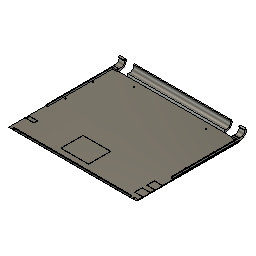
D_case (Autodesk Fusion 360 design; units mm, degrees)
Autodesk Fusion 360 part; units mm, degrees
sketch "Sketch2" plane through (0, 0, 0) normal (1, 0, 0) x (0, 0, -1)
  line L0 (0, 0) -> (0, 1.5)
  line L1 (0, 1.5) -> (190.1699, 1.5)
  line L2 (0, 0) -> (190.1699, 0)
  circle A0 centre (194.5, 12) radius 10.5
  circle A1 centre (194.5, 12) radius 9
  circle A2 centre (190.1699, 17.5) radius 17.5
  circle A3 centre (190.1699, 17.5) radius 16
  line L3 (203.5, 12) -> (205, 12)
  circle A4 centre (194.5, 12) radius 7.5
  line L4 (194.5, 12) -> (202.9853, 15)
  line L5 (194.5, 12) -> (190.1699, 1.5)
  dimension "d1" = 1.5
  dimension "d2" = 21
  dimension "d3" = 18
  dimension "d4" = 35
  dimension "d5" = 32
  dimension "d6" = 10.5
  dimension "d7" = 205
  dimension "d48" = 15
  dimension "d50" = 3
  constraint coincident L0.start L2.start
  constraint vertical L0
  constraint perpendicular L0 L1
  constraint perpendicular L0 L2
  constraint concentric A0 A1
  constraint tangent A0 A2
  constraint tangent L2 A2
  constraint coincident L2.end A2
  constraint concentric A2 A3
  constraint coincident L1.end A3
  constraint coincident A1 L3.start
  constraint coincident A0 L3.end
  constraint horizontal L3
  constraint tangent L1 A0
  constraint concentric A0 A4
  constraint coincident A0.centre A1.centre
  constraint coincident A1 L4.end
  measures "d1" distance of L0.start L0.end
  measures "d2" diameter of A0
  measures "d3" diameter of A1
  measures "d4" diameter of A2
  measures "d5" diameter of A3
  measures "d6" distance of L1 L3
  measures "d7" distance of L0 L3.end
  measures "d48" diameter of A4
  measures "d50" vertical distance of L3.start L4.end
extrude "Extrude1" add sketch "Sketch2" along normal blind 230.6 contours L0 L1 L2 A2 | L1 A0 A2 A3 | A0 A3 | A0 A3 L5 | A0 A1 A3 L5 | A0 A1 A3 L3 | A1 A4 L4 L5 picked at (191.2125, 0.5585) picked at (190.5457, 1.771) picked at (199.275, 4.984)
sketch "Sketch3" plane through (0, 0, 0) normal (0, -1, 0) x (1, 0, 0)
  line L0 (0, 0) -> (0, -190.1699)
  line L1 (0, -190.1699) -> (230.6, -190.1699)
  line L2 (230.6, -190.1699) -> (230.6, 0)
  line L3 (230.6, 0) -> (0, 0)
  circle A0 centre (6, -6) radius 6
  circle A1 centre (224.6, -6) radius 6
  line L4 (230.6, -6) -> (230.6, 0)
  line L5 (224.6, 0) -> (230.6, 0)
  line L6 (6, 0) -> (0, 0)
  line L7 (0, -6) -> (0, 0)
  dimension "d10" = 12
  dimension "d11" = 12
  constraint tangent L3 A0
  constraint tangent L0 A0
  constraint tangent L3 A1
  constraint tangent L2 A1
  constraint coincident A1 L4.start
  constraint coincident L2.end L3.start
  constraint tangent A1 L4
  constraint coincident A1 L5.start
  constraint tangent A1 L5
  constraint coincident A0 L6.start
  constraint coincident L0.start L3.end
  constraint perpendicular L0 L6
  constraint coincident A0 L7.start
  constraint perpendicular L6 L7
  measures "d10" diameter of A0
  measures "d11" diameter of A1
extrude "Extrude2" cut sketch "Sketch3" against normal through all contours L0 L3 A0 L6 L7 | L2 L3 A1 L4 L5
sketch "Sketch4" plane through (0, 0, 0) normal (0, -1, 0) x (1, 0, 0)
  arc A0 (6, 0) -> (0, -6) centre (6, -6) ccw
  line L0 (0, -6) -> (0, -190.1699)
  line L1 (0, -190.1699) -> (230.6, -190.1699)
  line L2 (230.6, -190.1699) -> (230.6, -6)
  arc A1 (230.6, -6) -> (224.6, 0) centre (224.6, -6) ccw
  line L3 (224.6, 0) -> (6, 0)
  line L4 (0, -190) -> (1.5, -190)
  line L5 (1.5, -190) -> (1.5, -215)
  line L6 (1.5, -215) -> (0, -215)
  line L7 (0, -215) -> (0, -190)
  line L8 (230.6, -190) -> (229.1, -190)
  line L9 (229.1, -190) -> (229.1, -215)
  line L10 (229.1, -215) -> (230.6, -215)
  line L11 (230.6, -215) -> (230.6, -190)
  line L12 (11.5, -190) -> (27.5, -190)
  line L13 (27.5, -190) -> (27.5, -215)
  line L14 (27.5, -215) -> (11.5, -215)
  line L15 (11.5, -215) -> (11.5, -190)
  line L16 (203.1, -190) -> (219.1, -190)
  line L17 (219.1, -190) -> (219.1, -215)
  line L18 (219.1, -215) -> (203.1, -215)
  line L19 (203.1, -215) -> (203.1, -190)
  dimension "d13" = 1.5
  dimension "d14" = 25
  dimension "d15" = 1.5
  dimension "d83" = 16
  dimension "d84" = 10
  dimension "d85" = 10
  dimension "d86" = 16
  dimension "d87" = 190
  constraint horizontal L4
  constraint vertical L5
  constraint horizontal L6
  constraint vertical L7
  constraint horizontal L8
  constraint vertical L9
  constraint horizontal L10
  constraint vertical L11
  constraint horizontal L12
  constraint vertical L13
  constraint horizontal L14
  constraint vertical L15
  constraint horizontal L16
  constraint vertical L17
  constraint horizontal L18
  constraint vertical L19
  constraint equal L5 L15
  constraint equal L13 L19
  constraint collinear L2 L11
  constraint collinear L0 L7
  constraint collinear L4 L12
  constraint collinear L12 L16
  constraint collinear L8 L16
  constraint equal L9 L17
  measures "d13" distance of L4.start L4.end
  measures "d14" distance of L4.start L6.end
  measures "d15" distance of L8.start L8.end
  measures "d83" distance of L13.end L14.end
  measures "d84" distance of L5 L15
  measures "d85" distance of L9 L17
  measures "d86" distance of L17.end L18.end
  measures "d87" distance of L3 L4
extrude "Extrude3" cut sketch "Sketch4" against normal through all contours L0 L1 L4 L5 L7 | L1 L5 L6 L7 | L1 L2 L8 L9 L11 | L1 L9 L10 L11 | L1 L12 L13 L15 | L1 L13 L14 L15 | L1 L17 L18 L19 | L1 L16 L17 L19
sketch "Sketch13" plane through (0, 1.5, 0) normal (0, 1, 0) x (-1, 0, 0)
  line L0 (0, -190) -> (0, -6)
  arc A0 (0, -6) -> (-6, 0) centre (-6, -6) ccw
  line L1 (-6, 0) -> (-224.6, 0)
  arc A1 (-224.6, 0) -> (-230.6, -6) centre (-224.6, -6) ccw
  line L2 (-230.6, -6) -> (-230.6, -190)
  line L3 (-230.6, -190) -> (-229.1, -190)
  line L4 (-229.1, -190) -> (-229.1, -190.1699)
  line L5 (-229.1, -190.1699) -> (-219.1, -190.1699)
  line L6 (-219.1, -190.1699) -> (-219.1, -190)
  line L7 (-219.1, -190) -> (-203.1, -190)
  line L8 (-203.1, -190) -> (-203.1, -190.1699)
  line L9 (-203.1, -190.1699) -> (-27.5, -190.1699)
  line L10 (-27.5, -190.1699) -> (-27.5, -190)
  line L11 (-27.5, -190) -> (-11.5, -190)
  line L12 (-11.5, -190) -> (-11.5, -190.1699)
  line L13 (-11.5, -190.1699) -> (-1.5, -190.1699)
  line L14 (-1.5, -190.1699) -> (-1.5, -190)
  line L15 (-1.5, -190) -> (0, -190)
  line L16 (-1.5, -188.1699) -> (-11.5, -188.1699)
  line L17 (-11.5, -188.1699) -> (-11.5, -192.1699)
  line L18 (-11.5, -192.1699) -> (-1.5, -192.1699)
  line L19 (-1.5, -192.1699) -> (-1.5, -188.1699)
  line L20 (-115.3, -219.4549) -> (-115.3, 20.5451) construction
  line L21 (-229.1, -188.1699) -> (-219.1, -188.1699)
  line L22 (-219.1, -188.1699) -> (-219.1, -192.1699)
  line L23 (-229.1, -192.1699) -> (-229.1, -188.1699)
  line L24 (-219.1, -192.1699) -> (-229.1, -192.1699)
  dimension "d90" = 2
  dimension "d91" = 4
  constraint horizontal L16
  constraint vertical L17
  constraint horizontal L18
  constraint vertical L19
  constraint collinear L12 L17
  constraint collinear L14 L19
  constraint perpendicular L1 L20
  constraint symmetric L16.start L20 L21.start
  constraint symmetric L16.end L20 L21.end
  constraint symmetric L17.end L20 L22.end
  constraint symmetric L18.end L20 L23.start
  measures "d90" distance of L13 L16
  measures "d91" distance of L16 L18
extrude "Extrude10" add sketch "Sketch13" along normal blind 3 contours L12 L13 L14 L16 L17 L19 | L13 L17 L18 L19 | L4 L5 L6 L21 L22 L23 | L5 L22 L23 L24
sketch "Sketch14" plane through (0, -50.4588, -17.8399) normal (0, 0.942809, 0.333333) x (1, 0, 0)
  line L0 (11.5, 194.8764) -> (11.5, 196.3764)
  line L1 (11.5, 196.3764) -> (1.5, 196.3764)
  line L2 (1.5, 196.3764) -> (1.5, 194.8764)
  line L3 (1.5, 194.8764) -> (11.5, 194.8764)
  line L4 (1.5, 196.3764) -> (11.5, 196.3764)
  line L5 (11.5, 196.3764) -> (11.5, 193.3764)
  line L6 (11.5, 193.3764) -> (1.5, 193.3764)
  line L7 (1.5, 193.3764) -> (1.5, 196.3764)
  line L8 (115.3, 222.5884) -> (115.3, -60) construction
  line L9 (0, 6.1569) -> (0, 179.6337)
  line L10 (230.6, 179.6337) -> (230.6, 6.1569)
  line L11 (229.1, 196.3764) -> (219.1, 196.3764)
  line L12 (219.1, 196.3764) -> (219.1, 193.3764)
  line L13 (219.1, 193.3764) -> (229.1, 193.3764)
  line L14 (229.1, 193.3764) -> (229.1, 196.3764)
  line L15 (1.5, 194.8764) -> (11.5, 194.8764)
  line L16 (229.1, 194.8764) -> (219.1, 194.8764)
  dimension "d94" = 3
  constraint horizontal L4
  constraint vertical L5
  constraint horizontal L6
  constraint vertical L7
  constraint coincident L1.end L2.start
  constraint collinear L0 L5
  constraint vertical L8
  constraint symmetric L8 L9 L10
  constraint symmetric L1.end L8 L11.start
  constraint symmetric L0.end L8 L11.end
  constraint symmetric L5.end L8 L12.end
  constraint symmetric L6.end L8 L13.end
  constraint coincident L2.end L3.start
  constraint coincident L0.start L3.end
  constraint symmetric L8 L2.end L16.start
  constraint symmetric L8 L0.start L16.end
  measures "d94" distance of L0.end L5.end
extrude "Extrude11" add sketch "Sketch14" against normal blind 2 contours L3 L5 L6 L7 L15 | L12 L13 L14 L16
sketch "Sketch5" plane through (230.6, 0, 0) normal (1, 0, 0) x (0, 0, -1)
  line L0 (190, 0) -> (190, 1.5)
  line L1 (190, 1.5) -> (6, 1.5)
  line L2 (6, 1.5) -> (6, 0)
  line L3 (6, 0) -> (190, 0)
  line L4 (15.8, 1.5) -> (29.3, 1.5)
  line L5 (29.3, 1.5) -> (29.3, 1)
  line L6 (29.3, 1) -> (15.8, 1)
  line L7 (15.8, 1) -> (15.8, 1.5)
  line L8 (37.8, 1.5) -> (51.3, 1.5)
  line L9 (51.3, 1.5) -> (51.3, 1)
  line L10 (51.3, 1) -> (37.8, 1)
  line L11 (37.8, 1) -> (37.8, 1.5)
  dimension "d18" = 13.5
  dimension "d19" = 13.5
  dimension "d20" = 22
  dimension "d21" = 9.8
  dimension "d22" = 0.5
  constraint horizontal L4
  constraint vertical L5
  constraint horizontal L6
  constraint vertical L7
  constraint coincident L1 L4.start
  constraint horizontal L8
  constraint vertical L9
  constraint horizontal L10
  constraint vertical L11
  constraint coincident L1 L8.start
  constraint collinear L6 L10
  measures "d18" distance of L5.end L6.end
  measures "d19" distance of L9.end L10.end
  measures "d20" distance of L5 L9
  measures "d21" distance of L2 L7
  measures "d22" distance of L4.start L6.end
extrude "Extrude4" cut sketch "Sketch5" against normal blind 15 contours L1 L8 L9 L10 L11 | L1 L4 L5 L6 L7
sketch "Sketch6" plane through (0, 0, 0) normal (-1, 0, 0) x (0, 0, 1)
  line L0 (-190, 1.5) -> (-190, 0)
  line L1 (-190, 0) -> (-6, 0)
  line L2 (-6, 0) -> (-6, 1.5)
  line L3 (-6, 1.5) -> (-190, 1.5)
  circle A0 centre (-36.6, 3.65) radius 2.75
  dimension "d25" = 2.15
  dimension "d26" = 30.6
  dimension "d27" = 5.5
  measures "d25" distance of L3 A0.centre
  measures "d26" distance of L2 A0.centre
  measures "d27" diameter of A0
extrude "Extrude5" cut sketch "Sketch6" against normal blind 3 contours L3 A0 picked at (-37.0583, 1.4228)
sketch "Sketch7" plane through (0, 1.5, 0) normal (0, 1, 0) x (-1, 0, 0)
  line L0 (0, -38.3146) -> (-3, -38.3146)
  line L1 (-3, -38.3146) -> (-3, -34.8854)
  line L2 (-3, -34.8854) -> (0, -34.8854)
  line L3 (0, -34.8854) -> (0, -6)
  arc A0 (0, -6) -> (-6, 0) centre (-6, -6) ccw
  line L4 (-6, 0) -> (-224.6, 0)
  arc A1 (-224.6, 0) -> (-230.6, -6) centre (-224.6, -6) ccw
  line L5 (-230.6, -6) -> (-230.6, -15.8)
  line L6 (-230.6, -15.8) -> (-215.6, -15.8)
  line L7 (-215.6, -15.8) -> (-215.6, -29.3)
  line L8 (-215.6, -29.3) -> (-230.6, -29.3)
  line L9 (-230.6, -29.3) -> (-230.6, -37.8)
  line L10 (-230.6, -37.8) -> (-215.6, -37.8)
  line L11 (-215.6, -37.8) -> (-215.6, -51.3)
  line L12 (-215.6, -51.3) -> (-230.6, -51.3)
  line L13 (0, -190) -> (0, -38.3146)
  line L14 (-1, -39.8146) -> (-16, -39.8146)
  line L15 (-16, -39.8146) -> (-16, -33.3146)
  line L16 (-16, -33.3146) -> (-1, -33.3146)
  line L17 (-1, -33.3146) -> (-1, -39.8146)
  line L18 (-80, -58) -> (-130, -58)
  line L19 (-130, -58) -> (-130, -18)
  line L20 (-130, -18) -> (-80, -18)
  line L21 (-80, -18) -> (-80, -58)
  line L22 (-230.6, -51.3) -> (-230.6, -190)
  line L23 (-230.6, -190) -> (-229.1, -190)
  line L24 (-229.1, -190) -> (-229.1, -188.1699)
  line L25 (-219.1, -188.1699) -> (-219.1, -190)
  line L26 (-219.1, -190) -> (-203.1, -190)
  line L27 (-203.1, -190) -> (-203.1, -190.1699)
  line L28 (-203.1, -190.1699) -> (-27.5, -190.1699)
  line L29 (-27.5, -190.1699) -> (-27.5, -190)
  line L30 (-27.5, -190) -> (-11.5, -190)
  line L31 (-11.5, -190) -> (-11.5, -188.1699)
  line L32 (-1.5, -188.1699) -> (-1.5, -190)
  line L33 (-1.5, -190) -> (0, -190)
  line L34 (-229.1, -188.1699) -> (-219.1, -188.1699)
  line L35 (-11.5, -188.1699) -> (-1.5, -188.1699)
  dimension "d30" = 15
  dimension "d31" = 6.5
  dimension "d32" = 1.5
  dimension "d33" = 1
  dimension "d34" = 80
  dimension "d35" = 50
  dimension "d36" = 40
  dimension "d37" = 18
  constraint horizontal L14
  constraint vertical L15
  constraint horizontal L16
  constraint vertical L17
  constraint horizontal L18
  constraint vertical L19
  constraint horizontal L20
  constraint vertical L21
  measures "d30" distance of L14.start L14.end
  measures "d31" distance of L14.end L15.end
  measures "d32" distance of L0 L14
  measures "d33" distance of L13 L17
  measures "d34" distance of L13 L21
  measures "d35" distance of L18.start L18.end
  measures "d36" distance of L18.end L19.end
  measures "d37" distance of L4 L20
extrude "Extrude6" cut sketch "Sketch7" against normal blind 0.5 contours L0 L1 L2 L14 L15 L16 L17 | L0 L1 L2 L17 | L18 L19 L20 L21
sketch "Sketch8" plane through (0, 1.5, 0) normal (0, 1, 0) x (-1, 0, 0)
  line L0 (-1, -33.3146) -> (-1, -34.8854)
  line L1 (-1, -34.8854) -> (0, -34.8854)
  line L2 (0, -34.8854) -> (0, -6)
  arc A0 (0, -6) -> (-6, 0) centre (-6, -6) ccw
  line L3 (-6, 0) -> (-224.6, 0)
  arc A1 (-224.6, 0) -> (-230.6, -6) centre (-224.6, -6) ccw
  line L4 (-230.6, -6) -> (-230.6, -15.8)
  line L5 (-230.6, -15.8) -> (-215.6, -15.8)
  line L6 (-215.6, -15.8) -> (-215.6, -29.3)
  line L7 (-215.6, -29.3) -> (-230.6, -29.3)
  line L8 (-230.6, -29.3) -> (-230.6, -37.8)
  line L9 (-230.6, -37.8) -> (-215.6, -37.8)
  line L10 (-215.6, -37.8) -> (-215.6, -51.3)
  line L11 (-215.6, -51.3) -> (-230.6, -51.3)
  line L12 (0, -190) -> (0, -38.3146)
  line L13 (0, -38.3146) -> (-1, -38.3146)
  line L14 (-1, -38.3146) -> (-1, -39.8146)
  line L15 (-1, -39.8146) -> (-16, -39.8146)
  line L16 (-16, -39.8146) -> (-16, -33.3146)
  line L17 (-16, -33.3146) -> (-1, -33.3146)
  line L18 (-130, -58) -> (-130, -18)
  line L19 (-130, -18) -> (-80, -18)
  line L20 (-80, -18) -> (-80, -58)
  line L21 (-80, -58) -> (-130, -58)
  line L22 (-1.5, -190.1699) -> (-3, -190.1699)
  line L23 (-3, -190.1699) -> (-3, -70.1699)
  line L24 (-3, -70.1699) -> (-1.5, -70.1699)
  line L25 (-1.5, -70.1699) -> (-1.5, -190.1699)
  line L26 (-229.1, -190.1699) -> (-227.6, -190.1699)
  line L27 (-227.6, -190.1699) -> (-227.6, -70.1699)
  line L28 (-227.6, -70.1699) -> (-229.1, -70.1699)
  line L29 (-229.1, -70.1699) -> (-229.1, -190.1699)
  line L30 (-10, -3.5) -> (-220.6, -3.5)
  line L31 (-220.6, -3.5) -> (-220.6, -5)
  line L32 (-220.6, -5) -> (-10, -5)
  line L33 (-10, -5) -> (-10, -3.5)
  line L34 (-230.6, -51.3) -> (-230.6, -190)
  line L35 (-230.6, -190) -> (-229.1, -190)
  line L36 (-229.1, -190) -> (-229.1, -188.1699)
  line L37 (-219.1, -188.1699) -> (-219.1, -190)
  line L38 (-219.1, -190) -> (-203.1, -190)
  line L39 (-203.1, -190) -> (-203.1, -190.1699)
  line L40 (-203.1, -190.1699) -> (-27.5, -190.1699)
  line L41 (-27.5, -190.1699) -> (-27.5, -190)
  line L42 (-27.5, -190) -> (-11.5, -190)
  line L43 (-11.5, -190) -> (-11.5, -188.1699)
  line L44 (-1.5, -188.1699) -> (-1.5, -190)
  line L45 (-1.5, -190) -> (0, -190)
  line L46 (-229.1, -188.1699) -> (-219.1, -188.1699)
  line L47 (-11.5, -188.1699) -> (-1.5, -188.1699)
  dimension "d40" = 120
  dimension "d41" = 1.5
  dimension "d42" = 1.5
  dimension "d43" = 120
  dimension "d44" = 1.5
  dimension "d45" = 3.5
  dimension "d64" = 10
  dimension "d65" = 10
  constraint horizontal L22
  constraint vertical L23
  constraint horizontal L24
  constraint vertical L25
  constraint horizontal L26
  constraint vertical L27
  constraint horizontal L28
  constraint vertical L29
  constraint horizontal L30
  constraint vertical L31
  constraint horizontal L32
  constraint vertical L33
  measures "d40" distance of L22.start L24.end
  measures "d41" distance of L23.end L24.end
  measures "d42" distance of L27.end L28.end
  measures "d43" distance of L26.end L27.end
  measures "d44" distance of L30.start L32.end
  measures "d45" distance of L3 L30
  measures "d64" distance of L2 L33
  measures "d65" distance of L4 L31
extrude "Extrude7" add sketch "Sketch8" along normal blind 3 contours L22 L23 L25 L44 L47 | L23 L24 L25 L47 | L26 L27 L29 L36 L46 | L27 L28 L29 L46 | L30 L31 L32 L33
sketch "Sketch9" plane through (0, 0, 0) normal (0, -1, 0) x (1, 0, 0)
  arc A0 (6, 0) -> (0, -6) centre (6, -6) ccw
  line L0 (0, -6) -> (0, -190)
  line L1 (0, -190) -> (1.5, -190)
  line L2 (219.1, -190.1699) -> (229.1, -190.1699)
  line L3 (229.1, -190) -> (230.6, -190)
  line L4 (230.6, -190) -> (230.6, -6)
  arc A1 (230.6, -6) -> (224.6, 0) centre (224.6, -6) ccw
  line L5 (224.6, 0) -> (6, 0)
  line L6 (115.3, 11.9246) -> (115.3, -196.6767) construction
  circle A2 centre (6, -7) radius 2
  circle A3 centre (224.6, -7) radius 2
  line L7 (203.1, -190) -> (219.1, -190)
  line L8 (219.1, -190) -> (219.1, -190.1699)
  line L9 (229.1, -190.1699) -> (229.1, -190)
  line L10 (1.5, -190) -> (1.5, -190.1699)
  line L11 (1.5, -190.1699) -> (11.5, -190.1699)
  line L12 (11.5, -190.1699) -> (11.5, -190)
  line L13 (11.5, -190) -> (27.5, -190)
  line L14 (27.5, -190) -> (27.5, -190.1699)
  line L15 (27.5, -190.1699) -> (203.1, -190.1699)
  line L16 (203.1, -190.1699) -> (203.1, -190)
  point P0 (6, -7)
  point P1 (6, -150)
  point P2 (6, -100)
  point P3 (224.6, -7)
  point P4 (224.6, -100)
  point P5 (224.6, -150)
  point P6 (50, -180)
  point P7 (180.6, -180)
  dimension "d53" = 6
  dimension "d54" = 7
  dimension "d55" = 6
  dimension "d56" = 100
  dimension "d57" = 150
  dimension "d58" = 6
  dimension "d70" = 4
  dimension "d88" = 180
  dimension "d89" = 44
  constraint perpendicular L2 L6
  constraint symmetric L0 L4 L6
  constraint symmetric P0 L6 P3
  constraint symmetric P1 L6 P5
  constraint symmetric P2 L6 P4
  constraint coincident P0 A2.centre
  constraint symmetric L6 A2 A3
  constraint symmetric L6 P6 P7
  measures "d53" distance of L0 P0
  measures "d54" distance of L5 P0
  measures "d55" distance of L0 P2
  measures "d56" distance of L5 P2
  measures "d57" distance of L5 P1
  measures "d58" distance of L0 P1
  measures "d70" diameter of A2
  measures "d88" distance of L5 P6
  measures "d89" horizontal distance of P1 P6
hole "Hole1" at (6, 0, -100) at (6, 0, -150) at (224.6, 0, -150) at (224.6, 0, -100) at (50, 0, -180) at (180.6, 0, -180) direction (0, 1, 0) diameter 2 depth 4 tip angle 118 countersink diameter 3.8 countersink angle 90
extrude "Extrude9" cut sketch "Sketch9" against normal blind 0.5 contours A2 | A3
sketch "Sketch11" plane through (0, 0.5, 0) normal (0, -1, 0) x (1, 0, 0)
  circle A0 centre (6, -7) radius 2
  point P0 (6, -7)
  constraint coincident P0 A0.centre
hole "Hole2" at (6, 0.5, -7) direction (0, 1, 0) diameter 2 depth 4 tip angle 118 countersink diameter 3.8 countersink angle 90
sketch "Sketch12" plane through (0, 0.5, 0) normal (0, -1, 0) x (1, 0, 0)
  circle A0 centre (224.6, -7) radius 2
  point P0 (224.6, -7)
  constraint coincident P0 A0.centre
hole "Hole3" at (224.6, 0.5, -7) direction (0, 1, 0) diameter 2 depth 4 tip angle 118 countersink diameter 3.8 countersink angle 90
sketch "Sketch10" plane through (0, 0, 0) normal (-1, 0, 0) x (0, 0, 1)
  arc A0 (-38.3146, 1.5) -> (-34.8854, 1.5) centre (-36.6, 3.65) ccw
  line L0 (-38.3146, 1.5) -> (-190, 1.5)
  line L1 (-190, 1.5) -> (-190, 0)
  line L2 (-190, 0) -> (-6, 0)
  line L3 (-6, 0) -> (-6, 1.5)
  line L4 (-6, 1.5) -> (-34.8854, 1.5)
  line L5 (-7.75, 0) -> (0, 0)
  line L6 (0, 0) -> (0, 7.75)
  circle A1 centre (-7.75, 7.75) radius 7.75
  dimension "d69" = 15.5
  constraint coincident L5.end L6.start
  constraint vertical L6
  constraint horizontal L5
  constraint coincident L5.start A1
  constraint tangent L5 A1
  constraint tangent L6 A1
  constraint coincident L6.end A1
  measures "d69" diameter of A1
extrude "Extrude8" cut sketch "Sketch10" against normal through all contours L3 L5 L6 A1 | L2 L3 L5 A1
